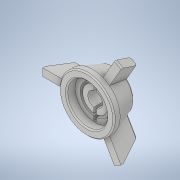
# Autodesk Inventor part: MINI-knob
Saved by Autodesk Inventor 2021 (Build 250183000, 183)
## iProperties
Created: 2019-11-28
Material: Všeobecné
Document SubType Name: Modeling
Density: 1 g/cm^3
Appearance: Výchozí
Project: ORIGINAL PRUSA MINI
Authority: Ing. Robert Turinský
Company: Prusa Development a.s.
Author: Ing. Robert Turinský
Title: MINI-knob
Revision Number: R4
Autodesk Inventor part; units mm, degrees
ref_plane "YZ Plane" through (0, 0, 0) normal (1, 0, 0) x (0, 1, 0)
ref_plane "XZ Plane" through (0, 0, 0) normal (0, 1, 0) x (-1, 0, 0)
ref_plane "XY Plane" through (0, 0, 0) normal (0, 0, 1) x (1, 0, 0)
sketch "Náčrt1" plane through (0, 0, 0) normal (0, 1, 0) x (-1, 0, 0)
  line L0 (0, -1.8) -> (0, 10.8) projected
  line L1 (24, 0) -> (-4, 0) projected
  line L2 (0, 0) -> (7, 0)
  line L3 (8, 0.95) -> (11, 9)
  line L4 (11, 9) -> (8, 9)
  line L5 (8, 9) -> (8, 8)
  line L6 (8, 8) -> (6, 8)
  line L7 (6, 8) -> (6, 1)
  line L8 (6, 1) -> (5, 1)
  line L9 (5, 1) -> (5, 8)
  line L10 (5, 8) -> (2.957, 8)
  line L11 (2.818, 0.95) -> (0, 0.95)
  line L12 (0, 0.95) -> (0, 0)
  line L13 (7, 0) -> (8, 0.95)
  line L14 (20, 9) -> (20, 8)
  line L15 (20, 8) -> (15, 0)
  line L16 (9.9328, 9) -> (7.1437, 1.5158)
  line L17 (7.1437, 1.5158) -> (5.5481, 0)
  line L18 (20, 9) -> (9.9328, 9)
  line L19 (5.5481, 0) -> (15, 0)
  line L20 (2.818, 0.95) -> (2.957, 8)
  line L21 (2.8279, 1.45) -> (0, 1.45)
  line L22 (0, 1.45) -> (0, 0.95)
  line L23 (2.8279, 1.45) -> (2.818, 0.95)
  dimension "d0" = 22
  dimension "d2" = 0.95
  dimension "d3" = 10
  dimension "d4" = 8
  dimension "d5" = 9
  dimension "d6" = 12
  dimension "d7" = 16
  dimension "d8" = 14
  dimension "d9" = 16
  dimension "d11" = 40
  dimension "d12" = 1
  dimension "d13" = 30
  dimension "d16" = 1
  dimension "d17" = 1
  dimension "d27" = 5.636
  dimension "d28" = 5.914
  dimension "d32" = 1
  dimension "d33" = 0.5
  constraints: 44 end point, 8 point on line, 5 perpendicular, 4 collinear, 4 parallel, 1 horizontal, 1 vertical
  measures "d0" diameter of L3.end L0
  measures "d2" distance between parallel lines of L1 L11
  measures "d3" diameter of L9 L0
  measures "d4" distance between parallel lines of L1 L10
  measures "d5" distance between parallel lines of L2 L4
  measures "d6" diameter of L7 L0
  measures "d7" diameter of L5 L0
  measures "d8" diameter of L2.end L0
  measures "d9" diameter of L3.start L0
  measures "d11" diameter of L14.start L0
  measures "d12" distance of L14.start L14.end
  measures "d13" diameter of L15.end L0
  measures "d16" distance between parallel lines of L3 L16
  measures "d17" distance between parallel lines of L13 L17
  measures "d27" diameter of L11.start L0
  measures "d28" diameter of L10.end L0
  measures "d32" distance between parallel lines of L1 L8
  measures "d33" distance between parallel lines of L11 L21
revolve "Rotace1" add sketch "Náčrt1" angle 360 about axis through (0, 0, -10) along (0, 0, 1) contours L0 L11 L20 L10 L9 L8 L7 L6 L5 L4 L16 L17 L1 | L17 L16 L4 L3 L13 L1
extrude "Vysunutí2" add sketch "Náčrt1" along normal mid plane 3 contours L17 L16 L4 L3 L13 L1 | L13 L3 L18 L14 L15 L1
pattern_circular "Kruhové pole1" count 3 over 360 about axis through (0, 0, -10) along (0, 0, 1) of "Vysunutí2"
sketch "Náčrt2" plane through (0, 0, 8) normal (0, 0, 1) x (1, 0, 0)
  circle A0 centre (0, 0) radius 8 projected
  circle A1 centre (0, 0) radius 6 projected
  circle A2 centre (0, 0) radius 5 projected
  line L0 (0, -15.4) -> (0, 15.4) projected
  line L1 (-15.4, 0) -> (15.4, 0) projected
  line L2 (0.5, 7.5) -> (-0.5, 7.5)
  line L3 (-0.5, 7.5) -> (-0.5, -7.5)
  line L4 (-0.5, -7.5) -> (0.5, -7.5)
  line L5 (0.5, -7.5) -> (0.5, 7.5)
  dimension "d23" = 15
  dimension "d24" = 1
  constraints: 8 end point, 2 parallel, 1 horizontal, 1 perpendicular, 2 other
  measures "d23" distance of L4.end L2.start
  measures "d24" distance of L2.start L2.end
extrude "Vysunutí3" cut sketch "Náčrt2" against normal up to surface (7.05 mm away) contours L2 L5 A1 L0 | L0 A1 L3 L2 | L4 L3 A1 L0 | L0 A1 L5 L4 | L5 A2 L0 A1 | A1 L0 A2 L5 | L0 A2 L3 A1 | A1 L3 A2 L0 | L5 L1 L0 A2 | A2 L0 L1 L5 | L0 L1 L3 A2 | A2 L3 L1 L0
chamfer "Zkosení1" distance 0.7 angle 45 6 edges at (-10.9187, -1.5, 0) (-10.9187, 1.5, 0) (4.1603, -10.2059, 0) (6.7584, -8.7059, 0) (4.1603, 10.2059, 0) (6.7584, 8.7059, 0)
revolve "Rotace2" add sketch "Náčrt1" angle 360 about axis through (0, 0, -10) along (0, 0, 1) contours L0 L21 L20 L11
sketch "Náčrt3" plane through (-20, 1.5, 9) normal (0, 0, 1) x (1, 0, 0)
  circle A0 centre (20, -1.5) radius 8 projected
  arc A1 (24.1496, 8.6873) -> (9.1028, 0) centre (20, -1.5) ccw projected
  line L0 (0, 0) -> (9.1028, 0) projected
  line L1 (0, -3) -> (0, 0) projected
  line L2 (9.1028, -3) -> (0, -3) projected
  arc A2 (9.1028, -3) -> (24.1496, -11.6873) centre (20, -1.5) ccw projected
  line L3 (28.701, -19.5705) -> (24.1496, -11.6873) projected
  line L4 (31.299, -18.0705) -> (28.701, -19.5705) projected
  line L5 (26.7477, -10.1873) -> (31.299, -18.0705) projected
  arc A3 (26.7477, -10.1873) -> (26.7477, 7.1873) centre (20, -1.5) ccw projected
  line L6 (31.299, 15.0705) -> (26.7477, 7.1873) projected
  line L7 (28.701, 16.5705) -> (31.299, 15.0705) projected
  line L8 (24.1496, 8.6873) -> (28.701, 16.5705) projected
  circle A4 centre (20, -1.5) radius 11
  constraints: 1 coincident, 3 other
extrude "Vysunutí4" add sketch "Náčrt3" along normal blind 2.45 contours A4 A3 A2 A1
chamfer "Zkosení2" distance 0.5 angle 45 2 edges at (-11, 0, 11.45) (-8, 0, 11.45)
equation "\"d17\" = d16"
